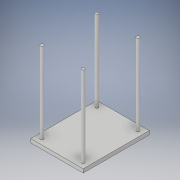
# Autodesk Inventor part: Relé - columnes
Saved by Autodesk Inventor 2019 (Build 230136000, 136)
## iProperties
Created: 2018-08-23
Part Number: Relé - columnes
Material: Genérico
Document SubType Name: Modeling
Designer: Albert Garangou Culebras
Density: 1 g/cm^3
Appearance: Valor por defecto
Author: Albert Garangou Culebras
Autodesk Inventor part; units mm, degrees
ref_plane "YZ Plane" through (0, 0, 0) normal (1, 0, 0) x (0, 1, 0)
ref_plane "XZ Plane" through (0, 0, 0) normal (0, 1, 0) x (-1, 0, 0)
ref_plane "XY Plane" through (0, 0, 0) normal (0, 0, 1) x (1, 0, 0)
sketch "Boceto1" plane through (0, 0, 0) normal (0, 1, 0) x (-1, 0, 0)
  line L0 (0, 0) -> (-42, 0)
  line L1 (-42, 0) -> (-42, -53)
  line L2 (-42, -53) -> (0, -53)
  line L3 (0, -53) -> (0, 0)
  circle A0 centre (-4.5, -4.5) radius 1.25
  circle A1 centre (-4.5, -48.5) radius 1.25
  circle A2 centre (-37.5, -48.5) radius 1.25
  circle A3 centre (-37.5, -4.5) radius 1.25
  line L4 (-36.25, -48.5) -> (-5.75, -48.5)
  line L5 (-4.5, -47.25) -> (-4.5, -5.75)
  line L6 (-5.75, -4.5) -> (-36.25, -4.5)
  line L7 (-37.5, -5.75) -> (-37.5, -47.25)
  dimension "d0" = 42
  dimension "d1" = 53
  dimension "d2" = 2.5
  dimension "d4" = 2.5
  dimension "d6" = 2.5
  dimension "d7" = 2.5
  constraints: 16 end point, 8 point on circle, 4 centre point, 3 horizontal, 2 parallel, 2 vertical, 1 perpendicular
  measures "d0" distance of L2.end L1.end
  measures "d1" distance of L1.end L0.end
  measures "d2" diameter of A0
  measures "d4" diameter of A1
  measures "d6" diameter of A2
  measures "d7" diameter of A3
extrude "Extrusión1" add sketch "Boceto1" along normal blind 3 contours L3 L2 L1 L0 | A0 | A0 L5 A1 L4 A2 L7 A3 L6 | A3 | A1 | A2
sketch "Boceto2" plane through (0, 3, 0) normal (0, 1, 0) x (1, 0, 0)
  circle A0 centre (4.5, 4.5) radius 1.25 projected
  circle A1 centre (4.5, 4.5) radius 1.25
  circle A2 centre (4.5, 48.5) radius 1.25 projected
  circle A3 centre (4.5, 48.5) radius 1.25
  circle A4 centre (37.5, 48.5) radius 1.25 projected
  circle A5 centre (37.5, 48.5) radius 1.25
  circle A6 centre (37.5, 4.5) radius 1.25 projected
  circle A7 centre (37.5, 4.5) radius 1.25
  point P0 (0, 0)
  constraints: 4 centre point, 4 coincident
extrude "Extrusión2" add sketch "Boceto2" along normal blind 65
